Autodesk Fusion 360 part; units mm, degrees
note: some values were not read from the file. Chosen so that the rebuilt part matches the saved one: which bodies a step acts on.
(part 2 of 2)
sketch "Sketch15" plane through (0, 0, 0.1) normal (0, 0, 1) x (1, 0, 0)
  line L0 (4.15, 10.85) -> (4.15, 6.55)
  line L1 (4.15, 6.55) -> (18.55, 6.55)
  line L2 (18.55, 6.55) -> (18.55, 10.85)
  line L3 (18.55, 10.85) -> (4.15, 10.85)
  line L4 (4.7609, 8.6617) -> (4.7609, 10.2617)
  line L5 (4.7609, 10.2617) -> (5.2444, 10.2617)
  line L6 (5.2444, 10.2617) -> (5.5347, 9.1703)
  line L7 (5.5347, 9.1703) -> (5.8218, 10.2617)
  line L8 (5.8218, 10.2617) -> (6.3063, 10.2617)
  line L9 (6.3063, 10.2617) -> (6.3063, 8.6617)
  line L10 (6.3063, 8.6617) -> (6.0062, 8.6617)
  line L11 (6.0062, 8.6617) -> (6.0062, 9.9212)
  line L12 (6.0062, 9.9212) -> (5.6886, 8.6617)
  line L13 (5.6886, 8.6617) -> (5.3776, 8.6617)
  line L14 (5.3776, 8.6617) -> (5.0611, 9.9212)
  line L15 (5.0611, 9.9212) -> (5.0611, 8.6617)
  line L16 (5.0611, 8.6617) -> (4.7609, 8.6617)
  line L17 (6.6872, 9.9779) -> (6.6872, 10.2617)
  line L18 (6.6872, 10.2617) -> (6.9939, 10.2617)
  line L19 (6.9939, 10.2617) -> (6.9939, 9.9779)
  line L20 (6.9939, 9.9779) -> (6.6872, 9.9779)
  line L21 (6.6872, 8.6617) -> (6.6872, 9.8207)
  line L22 (6.6872, 9.8207) -> (6.9939, 9.8207)
  line L23 (6.9939, 9.8207) -> (6.9939, 8.6617)
  line L24 (6.9939, 8.6617) -> (6.6872, 8.6617)
  line L25 (8.381, 9.478) -> (8.0787, 9.4235)
  spline S0 degree 2 poles (8.0787, 9.4235) (8.0634, 9.5141) (8.0088, 9.5599) knots 0 0 0 1 1 1
  spline S1 degree 2 poles (8.0088, 9.5599) (7.9553, 9.6057) (7.8691, 9.6057) knots 0 0 0 1 1 1
  spline S2 degree 2 poles (7.8691, 9.6057) (7.7545, 9.6057) (7.6858, 9.5261) knots 0 0 0 1 1 1
  spline S3 degree 2 poles (7.6858, 9.5261) (7.6181, 9.4475) (7.6181, 9.2619) knots 0 0 0 1 1 1
  spline S4 degree 2 poles (7.6181, 9.2619) (7.6181, 9.0557) (7.6869, 8.9705) knots 0 0 0 1 1 1
  spline S5 degree 2 poles (7.6869, 8.9705) (7.7567, 8.8854) (7.8735, 8.8854) knots 0 0 0 1 1 1
  spline S6 degree 2 poles (7.8735, 8.8854) (7.9608, 8.8854) (8.0165, 8.9345) knots 0 0 0 1 1 1
  spline S7 degree 2 poles (8.0165, 8.9345) (8.0721, 8.9847) (8.095, 9.1059) knots 0 0 0 1 1 1
  line L26 (8.095, 9.1059) -> (8.3963, 9.0546)
  spline S8 degree 2 poles (8.3963, 9.0546) (8.3493, 8.8472) (8.2162, 8.7413) knots 0 0 0 1 1 1
  spline S9 degree 2 poles (8.2162, 8.7413) (8.083, 8.6355) (7.8593, 8.6355) knots 0 0 0 1 1 1
  spline S10 degree 2 poles (7.8593, 8.6355) (7.605, 8.6355) (7.4533, 8.7959) knots 0 0 0 1 1 1
  spline S11 degree 2 poles (7.4533, 8.7959) (7.3027, 8.9564) (7.3027, 9.2401) knots 0 0 0 1 1 1
  spline S12 degree 2 poles (7.3027, 9.2401) (7.3027, 9.5272) (7.4544, 9.6865) knots 0 0 0 1 1 1
  spline S13 degree 2 poles (7.4544, 9.6865) (7.6061, 9.8469) (7.8648, 9.8469) knots 0 0 0 1 1 1
  spline S14 degree 2 poles (7.8648, 9.8469) (8.0765, 9.8469) (8.2009, 9.7553) knots 0 0 0 1 1 1
  spline S15 degree 2 poles (8.2009, 9.7553) (8.3264, 9.6647) (8.381, 9.478) knots 0 0 0 1 1 1
  line L27 (8.9692, 8.6617) -> (8.6625, 8.6617)
  line L28 (8.6625, 8.6617) -> (8.6625, 9.8207)
  line L29 (8.6625, 9.8207) -> (8.9474, 9.8207)
  line L30 (8.9474, 9.8207) -> (8.9474, 9.6559)
  spline S16 degree 2 poles (8.9474, 9.6559) (9.0205, 9.7727) (9.0783, 9.8098) knots 0 0 0 1 1 1
  spline S17 degree 2 poles (9.0783, 9.8098) (9.1373, 9.8469) (9.2115, 9.8469) knots 0 0 0 1 1 1
  spline S18 degree 2 poles (9.2115, 9.8469) (9.3163, 9.8469) (9.4134, 9.7891) knots 0 0 0 1 1 1
  line L31 (9.4134, 9.7891) -> (9.3185, 9.5217)
  spline S19 degree 2 poles (9.3185, 9.5217) (9.241, 9.5719) (9.1744, 9.5719) knots 0 0 0 1 1 1
  spline S20 degree 2 poles (9.1744, 9.5719) (9.11, 9.5719) (9.0653, 9.5359) knots 0 0 0 1 1 1
  spline S21 degree 2 poles (9.0653, 9.5359) (9.0205, 9.501) (8.9943, 9.4082) knots 0 0 0 1 1 1
  spline S22 degree 2 poles (8.9943, 9.4082) (8.9692, 9.3154) (8.9692, 9.0197) knots 0 0 0 1 1 1
  line L32 (8.9692, 9.0197) -> (8.9692, 8.6617)
  spline S23 degree 2 poles (9.5367, 9.2576) (9.5367, 9.4104) (9.612, 9.5534) knots 0 0 0 1 1 1
  spline S24 degree 2 poles (9.612, 9.5534) (9.6873, 9.6963) (9.8248, 9.7716) knots 0 0 0 1 1 1
  spline S25 degree 2 poles (9.8248, 9.7716) (9.9634, 9.8469) (10.1337, 9.8469) knots 0 0 0 1 1 1
  spline S26 degree 2 poles (10.1337, 9.8469) (10.3967, 9.8469) (10.5648, 9.6756) knots 0 0 0 1 1 1
  spline S27 degree 2 poles (10.5648, 9.6756) (10.7329, 9.5053) (10.7329, 9.2445) knots 0 0 0 1 1 1
  spline S28 degree 2 poles (10.7329, 9.2445) (10.7329, 8.9815) (10.5626, 8.8079) knots 0 0 0 1 1 1
  spline S29 degree 2 poles (10.5626, 8.8079) (10.3934, 8.6355) (10.1359, 8.6355) knots 0 0 0 1 1 1
  spline S30 degree 2 poles (10.1359, 8.6355) (9.9765, 8.6355) (9.8314, 8.7075) knots 0 0 0 1 1 1
  spline S31 degree 2 poles (9.8314, 8.7075) (9.6873, 8.7795) (9.612, 8.9182) knots 0 0 0 1 1 1
  spline S32 degree 2 poles (9.612, 8.9182) (9.5367, 9.0579) (9.5367, 9.2576) knots 0 0 0 1 1 1
  spline S33 degree 2 poles (9.851, 9.2412) (9.851, 9.0688) (9.9329, 8.9771) knots 0 0 0 1 1 1
  spline S34 degree 2 poles (9.9329, 8.9771) (10.0147, 8.8854) (10.1348, 8.8854) knots 0 0 0 1 1 1
  spline S35 degree 2 poles (10.1348, 8.8854) (10.2548, 8.8854) (10.3356, 8.9771) knots 0 0 0 1 1 1
  spline S36 degree 2 poles (10.3356, 8.9771) (10.4174, 9.0688) (10.4174, 9.2434) knots 0 0 0 1 1 1
  spline S37 degree 2 poles (10.4174, 9.2434) (10.4174, 9.4137) (10.3356, 9.5053) knots 0 0 0 1 1 1
  spline S38 degree 2 poles (10.3356, 9.5053) (10.2548, 9.597) (10.1348, 9.597) knots 0 0 0 1 1 1
  spline S39 degree 2 poles (10.1348, 9.597) (10.0147, 9.597) (9.9329, 9.5053) knots 0 0 0 1 1 1
  spline S40 degree 2 poles (9.9329, 9.5053) (9.851, 9.4137) (9.851, 9.2412) knots 0 0 0 1 1 1
  line L33 (11.6386, 9.1823) -> (11.9529, 9.2128)
  spline S41 degree 2 poles (11.9529, 9.2128) (11.9813, 9.0546) (12.0675, 8.9804) knots 0 0 0 1 1 1
  spline S42 degree 2 poles (12.0675, 8.9804) (12.1549, 8.9062) (12.3022, 8.9062) knots 0 0 0 1 1 1
  spline S43 degree 2 poles (12.3022, 8.9062) (12.4583, 8.9062) (12.5368, 8.9716) knots 0 0 0 1 1 1
  spline S44 degree 2 poles (12.5368, 8.9716) (12.6165, 9.0382) (12.6165, 9.1266) knots 0 0 0 1 1 1
  spline S45 degree 2 poles (12.6165, 9.1266) (12.6165, 9.1834) (12.5827, 9.2227) knots 0 0 0 1 1 1
  spline S46 degree 2 poles (12.5827, 9.2227) (12.5499, 9.263) (12.467, 9.2925) knots 0 0 0 1 1 1
  spline S47 degree 2 poles (12.467, 9.2925) (12.4102, 9.3122) (12.2083, 9.3624) knots 0 0 0 1 1 1
  spline S48 degree 2 poles (12.2083, 9.3624) (11.9486, 9.4268) (11.8438, 9.5206) knots 0 0 0 1 1 1
  spline S49 degree 2 poles (11.8438, 9.5206) (11.6965, 9.6527) (11.6965, 9.8426) knots 0 0 0 1 1 1
  spline S50 degree 2 poles (11.6965, 9.8426) (11.6965, 9.9648) (11.7652, 10.0707) knots 0 0 0 1 1 1
  spline S51 degree 2 poles (11.7652, 10.0707) (11.8351, 10.1776) (11.965, 10.2333) knots 0 0 0 1 1 1
  spline S52 degree 2 poles (11.965, 10.2333) (12.0959, 10.289) (12.2804, 10.289) knots 0 0 0 1 1 1
  spline S53 degree 2 poles (12.2804, 10.289) (12.5816, 10.289) (12.7333, 10.1569) knots 0 0 0 1 1 1
  spline S54 degree 2 poles (12.7333, 10.1569) (12.8861, 10.0248) (12.8937, 9.8044) knots 0 0 0 1 1 1
  line L34 (12.8937, 9.8044) -> (12.5707, 9.7902)
  spline S55 degree 2 poles (12.5707, 9.7902) (12.5499, 9.9135) (12.4812, 9.967) knots 0 0 0 1 1 1
  spline S56 degree 2 poles (12.4812, 9.967) (12.4135, 10.0216) (12.2771, 10.0216) knots 0 0 0 1 1 1
  spline S57 degree 2 poles (12.2771, 10.0216) (12.1363, 10.0216) (12.0566, 9.9637) knots 0 0 0 1 1 1
  spline S58 degree 2 poles (12.0566, 9.9637) (12.0053, 9.9266) (12.0053, 9.8644) knots 0 0 0 1 1 1
  spline S59 degree 2 poles (12.0053, 9.8644) (12.0053, 9.8077) (12.0534, 9.7673) knots 0 0 0 1 1 1
  spline S60 degree 2 poles (12.0534, 9.7673) (12.1145, 9.716) (12.3502, 9.6603) knots 0 0 0 1 1 1
  spline S61 degree 2 poles (12.3502, 9.6603) (12.586, 9.6046) (12.6984, 9.5446) knots 0 0 0 1 1 1
  spline S62 degree 2 poles (12.6984, 9.5446) (12.8119, 9.4857) (12.8752, 9.382) knots 0 0 0 1 1 1
  spline S63 degree 2 poles (12.8752, 9.382) (12.9396, 9.2794) (12.9396, 9.1277) knots 0 0 0 1 1 1
  spline S64 degree 2 poles (12.9396, 9.1277) (12.9396, 8.9902) (12.8632, 8.8701) knots 0 0 0 1 1 1
  spline S65 degree 2 poles (12.8632, 8.8701) (12.7868, 8.7501) (12.6471, 8.6911) knots 0 0 0 1 1 1
  spline S66 degree 2 poles (12.6471, 8.6911) (12.5074, 8.6333) (12.2989, 8.6333) knots 0 0 0 1 1 1
  spline S67 degree 2 poles (12.2989, 8.6333) (11.9955, 8.6333) (11.8329, 8.773) knots 0 0 0 1 1 1
  spline S68 degree 2 poles (11.8329, 8.773) (11.6703, 8.9138) (11.6386, 9.1823) knots 0 0 0 1 1 1
  line L35 (13.9425, 9.0306) -> (14.2481, 8.9793)
  spline S69 degree 2 poles (14.2481, 8.9793) (14.1892, 8.8112) (14.0615, 8.7228) knots 0 0 0 1 1 1
  spline S70 degree 2 poles (14.0615, 8.7228) (13.9349, 8.6355) (13.7439, 8.6355) knots 0 0 0 1 1 1
  spline S71 degree 2 poles (13.7439, 8.6355) (13.4416, 8.6355) (13.2964, 8.833) knots 0 0 0 1 1 1
  spline S72 degree 2 poles (13.2964, 8.833) (13.1818, 8.9913) (13.1818, 9.2325) knots 0 0 0 1 1 1
  spline S73 degree 2 poles (13.1818, 9.2325) (13.1818, 9.5206) (13.3324, 9.6832) knots 0 0 0 1 1 1
  spline S74 degree 2 poles (13.3324, 9.6832) (13.483, 9.8469) (13.7133, 9.8469) knots 0 0 0 1 1 1
  spline S75 degree 2 poles (13.7133, 9.8469) (13.972, 9.8469) (14.1215, 9.6756) knots 0 0 0 1 1 1
  spline S76 degree 2 poles (14.1215, 9.6756) (14.271, 9.5053) (14.2645, 9.1528) knots 0 0 0 1 1 1
  line L36 (14.2645, 9.1528) -> (13.4961, 9.1528)
  spline S77 degree 2 poles (13.4961, 9.1528) (13.4994, 9.0164) (13.5704, 8.94) knots 0 0 0 1 1 1
  spline S78 degree 2 poles (13.5704, 8.94) (13.6413, 8.8647) (13.7472, 8.8647) knots 0 0 0 1 1 1
  spline S79 degree 2 poles (13.7472, 8.8647) (13.8192, 8.8647) (13.8683, 8.904) knots 0 0 0 1 1 1
  spline S80 degree 2 poles (13.8683, 8.904) (13.9174, 8.9433) (13.9425, 9.0306) knots 0 0 0 1 1 1
  spline S81 degree 2 poles (13.96, 9.3405) (13.9567, 9.4737) (13.8912, 9.5424) knots 0 0 0 1 1 1
  spline S82 degree 2 poles (13.8912, 9.5424) (13.8257, 9.6123) (13.7319, 9.6123) knots 0 0 0 1 1 1
  spline S83 degree 2 poles (13.7319, 9.6123) (13.6315, 9.6123) (13.566, 9.5392) knots 0 0 0 1 1 1
  spline S84 degree 2 poles (13.566, 9.5392) (13.5005, 9.466) (13.5016, 9.3405) knots 0 0 0 1 1 1
  line L37 (13.5016, 9.3405) -> (13.96, 9.3405)
  line L38 (14.8702, 8.6617) -> (14.5635, 8.6617)
  line L39 (14.5635, 8.6617) -> (14.5635, 9.8207)
  line L40 (14.5635, 9.8207) -> (14.8483, 9.8207)
  line L41 (14.8483, 9.8207) -> (14.8483, 9.6559)
  spline S85 degree 2 poles (14.8483, 9.6559) (14.9215, 9.7727) (14.9793, 9.8098) knots 0 0 0 1 1 1
  spline S86 degree 2 poles (14.9793, 9.8098) (15.0382, 9.8469) (15.1125, 9.8469) knots 0 0 0 1 1 1
  spline S87 degree 2 poles (15.1125, 9.8469) (15.2172, 9.8469) (15.3144, 9.7891) knots 0 0 0 1 1 1
  line L42 (15.3144, 9.7891) -> (15.2194, 9.5217)
  spline S88 degree 2 poles (15.2194, 9.5217) (15.1419, 9.5719) (15.0753, 9.5719) knots 0 0 0 1 1 1
  spline S89 degree 2 poles (15.0753, 9.5719) (15.011, 9.5719) (14.9662, 9.5359) knots 0 0 0 1 1 1
  spline S90 degree 2 poles (14.9662, 9.5359) (14.9215, 9.501) (14.8953, 9.4082) knots 0 0 0 1 1 1
  spline S91 degree 2 poles (14.8953, 9.4082) (14.8702, 9.3154) (14.8702, 9.0197) knots 0 0 0 1 1 1
  line L43 (14.8702, 9.0197) -> (14.8702, 8.6617)
  line L44 (15.8273, 8.6617) -> (15.3601, 9.8207)
  line L45 (15.3601, 9.8207) -> (15.6821, 9.8207)
  line L46 (15.6821, 9.8207) -> (15.9004, 9.2292)
  line L47 (15.9004, 9.2292) -> (15.9637, 9.0317)
  spline S92 degree 2 poles (15.9637, 9.0317) (15.9888, 9.107) (15.9953, 9.131) knots 0 0 0 1 1 1
  spline S93 degree 2 poles (15.9953, 9.131) (16.0106, 9.1801) (16.0281, 9.2292) knots 0 0 0 1 1 1
  line L48 (16.0281, 9.2292) -> (16.2486, 9.8207)
  line L49 (16.2486, 9.8207) -> (16.564, 9.8207)
  line L50 (16.564, 9.8207) -> (16.1034, 8.6617)
  line L51 (16.1034, 8.6617) -> (15.8273, 8.6617)
  spline S94 degree 2 poles (16.7429, 9.2576) (16.7429, 9.4104) (16.8182, 9.5534) knots 0 0 0 1 1 1
  spline S95 degree 2 poles (16.8182, 9.5534) (16.8935, 9.6963) (17.031, 9.7716) knots 0 0 0 1 1 1
  spline S96 degree 2 poles (17.031, 9.7716) (17.1696, 9.8469) (17.3399, 9.8469) knots 0 0 0 1 1 1
  spline S97 degree 2 poles (17.3399, 9.8469) (17.6029, 9.8469) (17.771, 9.6756) knots 0 0 0 1 1 1
  spline S98 degree 2 poles (17.771, 9.6756) (17.9391, 9.5053) (17.9391, 9.2445) knots 0 0 0 1 1 1
  spline S99 degree 2 poles (17.9391, 9.2445) (17.9391, 8.9815) (17.7688, 8.8079) knots 0 0 0 1 1 1
  spline S100 degree 2 poles (17.7688, 8.8079) (17.5997, 8.6355) (17.3421, 8.6355) knots 0 0 0 1 1 1
  spline S101 degree 2 poles (17.3421, 8.6355) (17.1827, 8.6355) (17.0376, 8.7075) knots 0 0 0 1 1 1
  spline S102 degree 2 poles (17.0376, 8.7075) (16.8935, 8.7795) (16.8182, 8.9182) knots 0 0 0 1 1 1
  spline S103 degree 2 poles (16.8182, 8.9182) (16.7429, 9.0579) (16.7429, 9.2576) knots 0 0 0 1 1 1
  spline S104 degree 2 poles (17.0572, 9.2412) (17.0572, 9.0688) (17.1391, 8.9771) knots 0 0 0 1 1 1
  spline S105 degree 2 poles (17.1391, 8.9771) (17.2209, 8.8854) (17.341, 8.8854) knots 0 0 0 1 1 1
  spline S106 degree 2 poles (17.341, 8.8854) (17.4611, 8.8854) (17.5418, 8.9771) knots 0 0 0 1 1 1
  spline S107 degree 2 poles (17.5418, 8.9771) (17.6237, 9.0688) (17.6237, 9.2434) knots 0 0 0 1 1 1
  spline S108 degree 2 poles (17.6237, 9.2434) (17.6237, 9.4137) (17.5418, 9.5053) knots 0 0 0 1 1 1
  spline S109 degree 2 poles (17.5418, 9.5053) (17.4611, 9.597) (17.341, 9.597) knots 0 0 0 1 1 1
  spline S110 degree 2 poles (17.341, 9.597) (17.2209, 9.597) (17.1391, 9.5053) knots 0 0 0 1 1 1
  spline S111 degree 2 poles (17.1391, 9.5053) (17.0572, 9.4137) (17.0572, 9.2412) knots 0 0 0 1 1 1
  line L52 (10.4517, 7.1524) -> (10.6743, 7.177)
  spline S112 degree 2 poles (10.6743, 7.177) (10.6825, 7.109) (10.7169, 7.0763) knots 0 0 0 1 1 1
  spline S113 degree 2 poles (10.7169, 7.0763) (10.7512, 7.0435) (10.8077, 7.0435) knots 0 0 0 1 1 1
  spline S114 degree 2 poles (10.8077, 7.0435) (10.8789, 7.0435) (10.9289, 7.109) knots 0 0 0 1 1 1
  spline S115 degree 2 poles (10.9289, 7.109) (10.9788, 7.1745) (10.9927, 7.3808) knots 0 0 0 1 1 1
  spline S116 degree 2 poles (10.9927, 7.3808) (10.906, 7.2801) (10.7758, 7.2801) knots 0 0 0 1 1 1
  spline S117 degree 2 poles (10.7758, 7.2801) (10.6342, 7.2801) (10.5311, 7.389) knots 0 0 0 1 1 1
  spline S118 degree 2 poles (10.5311, 7.389) (10.4287, 7.4986) (10.4287, 7.6738) knots 0 0 0 1 1 1
  spline S119 degree 2 poles (10.4287, 7.6738) (10.4287, 7.8564) (10.5368, 7.9677) knots 0 0 0 1 1 1
  spline S120 degree 2 poles (10.5368, 7.9677) (10.6457, 8.0798) (10.8135, 8.0798) knots 0 0 0 1 1 1
  spline S121 degree 2 poles (10.8135, 8.0798) (10.996, 8.0798) (11.113, 7.9382) knots 0 0 0 1 1 1
  spline S122 degree 2 poles (11.113, 7.9382) (11.2301, 7.7974) (11.2301, 7.4741) knots 0 0 0 1 1 1
  spline S123 degree 2 poles (11.2301, 7.4741) (11.2301, 7.145) (11.1081, 6.9993) knots 0 0 0 1 1 1
  spline S124 degree 2 poles (11.1081, 6.9993) (10.9862, 6.8536) (10.7905, 6.8536) knots 0 0 0 1 1 1
  spline S125 degree 2 poles (10.7905, 6.8536) (10.6497, 6.8536) (10.563, 6.9281) knots 0 0 0 1 1 1
  spline S126 degree 2 poles (10.563, 6.9281) (10.4762, 7.0034) (10.4517, 7.1524) knots 0 0 0 1 1 1
  spline S127 degree 2 poles (10.9723, 7.655) (10.9723, 7.7663) (10.9207, 7.8277) knots 0 0 0 1 1 1
  spline S128 degree 2 poles (10.9207, 7.8277) (10.8699, 7.8891) (10.8028, 7.8891) knots 0 0 0 1 1 1
  spline S129 degree 2 poles (10.8028, 7.8891) (10.739, 7.8891) (10.6964, 7.8383) knots 0 0 0 1 1 1
  spline S130 degree 2 poles (10.6964, 7.8383) (10.6547, 7.7884) (10.6547, 7.6738) knots 0 0 0 1 1 1
  spline S131 degree 2 poles (10.6547, 7.6738) (10.6547, 7.5576) (10.7005, 7.5027) knots 0 0 0 1 1 1
  spline S132 degree 2 poles (10.7005, 7.5027) (10.7463, 7.4487) (10.8151, 7.4487) knots 0 0 0 1 1 1
  spline S133 degree 2 poles (10.8151, 7.4487) (10.8814, 7.4487) (10.9264, 7.5011) knots 0 0 0 1 1 1
  spline S134 degree 2 poles (10.9264, 7.5011) (10.9723, 7.5535) (10.9723, 7.655) knots 0 0 0 1 1 1
  line L53 (11.4535, 6.8176) -> (11.7163, 6.7857)
  spline S135 degree 2 poles (11.7163, 6.7857) (11.7228, 6.7398) (11.7466, 6.7227) knots 0 0 0 1 1 1
  spline S136 degree 2 poles (11.7466, 6.7227) (11.7793, 6.6981) (11.8497, 6.6981) knots 0 0 0 1 1 1
  spline S137 degree 2 poles (11.8497, 6.6981) (11.9397, 6.6981) (11.9848, 6.7251) knots 0 0 0 1 1 1
  spline S138 degree 2 poles (11.9848, 6.7251) (12.0151, 6.7431) (12.0306, 6.7832) knots 0 0 0 1 1 1
  spline S139 degree 2 poles (12.0306, 6.7832) (12.0412, 6.8119) (12.0412, 6.8888) knots 0 0 0 1 1 1
  line L54 (12.0412, 6.8888) -> (12.0412, 7.0157)
  spline S140 degree 2 poles (12.0412, 7.0157) (11.9381, 6.8749) (11.7809, 6.8749) knots 0 0 0 1 1 1
  spline S141 degree 2 poles (11.7809, 6.8749) (11.6058, 6.8749) (11.5035, 7.0231) knots 0 0 0 1 1 1
  spline S142 degree 2 poles (11.5035, 7.0231) (11.4232, 7.1401) (11.4232, 7.3145) knots 0 0 0 1 1 1
  spline S143 degree 2 poles (11.4232, 7.3145) (11.4232, 7.533) (11.528, 7.6484) knots 0 0 0 1 1 1
  spline S144 degree 2 poles (11.528, 7.6484) (11.6336, 7.7639) (11.79, 7.7639) knots 0 0 0 1 1 1
  spline S145 degree 2 poles (11.79, 7.7639) (11.9512, 7.7639) (12.056, 7.6222) knots 0 0 0 1 1 1
  line L55 (12.056, 7.6222) -> (12.056, 7.7442)
  line L56 (12.056, 7.7442) -> (12.2713, 7.7442)
  line L57 (12.2713, 7.7442) -> (12.2713, 6.9641)
  spline S146 degree 2 poles (12.2713, 6.9641) (12.2713, 6.8102) (12.2459, 6.7341) knots 0 0 0 1 1 1
  spline S147 degree 2 poles (12.2459, 6.7341) (12.2205, 6.658) (12.1747, 6.6146) knots 0 0 0 1 1 1
  spline S148 degree 2 poles (12.1747, 6.6146) (12.1288, 6.5712) (12.0519, 6.5467) knots 0 0 0 1 1 1
  spline S149 degree 2 poles (12.0519, 6.5467) (11.9758, 6.5221) (11.8587, 6.5221) knots 0 0 0 1 1 1
  spline S150 degree 2 poles (11.8587, 6.5221) (11.6377, 6.5221) (11.5452, 6.5982) knots 0 0 0 1 1 1
  spline S151 degree 2 poles (11.5452, 6.5982) (11.4527, 6.6735) (11.4527, 6.7898) knots 0 0 0 1 1 1
  spline S152 degree 2 poles (11.4527, 6.7898) (11.4527, 6.8012) (11.4535, 6.8176) knots 0 0 0 1 1 1
  spline S153 degree 2 poles (11.659, 7.3276) (11.659, 7.1892) (11.7122, 7.1246) knots 0 0 0 1 1 1
  spline S154 degree 2 poles (11.7122, 7.1246) (11.7662, 7.0607) (11.8448, 7.0607) knots 0 0 0 1 1 1
  spline S155 degree 2 poles (11.8448, 7.0607) (11.9291, 7.0607) (11.9872, 7.1262) knots 0 0 0 1 1 1
  spline S156 degree 2 poles (11.9872, 7.1262) (12.0453, 7.1925) (12.0453, 7.3218) knots 0 0 0 1 1 1
  spline S157 degree 2 poles (12.0453, 7.3218) (12.0453, 7.4569) (11.9897, 7.5224) knots 0 0 0 1 1 1
  spline S158 degree 2 poles (11.9897, 7.5224) (11.934, 7.5879) (11.8489, 7.5879) knots 0 0 0 1 1 1
  spline S159 degree 2 poles (11.8489, 7.5879) (11.7662, 7.5879) (11.7122, 7.5232) knots 0 0 0 1 1 1
  spline S160 degree 2 poles (11.7122, 7.5232) (11.659, 7.4594) (11.659, 7.3276) knots 0 0 0 1 1 1
extrude "Extrude15" cut sketch "Sketch15" against normal blind 0.05 contours L1 L53 S135 S136 S137 S138 S139 L54 S140 S141 S142 S143 S144 S145 L55 L56 L57 S146 S147 S148 S150 S151 S152 | L4 L5 L6 L7 L8 L9 L10 L11 L12 L13 L14 L15 L16 | L17 L18 L19 L20 | L21 L22 L23 L24 | L25 S0 S1 S2 S3 S4 S5 S6 S7 L26 S8 S9 S10 S11 S12 S13 S14 S15 | L27 L28 L29 L30 S16 S17 S18 L31 S19 S20 S21 S22 L32 | S23 S24 S25 S26 S27 S28 S29 S30 S31 S32 | L33 S41 S42 S43 S44 S45 S46 S47 S48 S49 S50 S51 S52 S53 S54 L34 S55 S56 S57 S58 S59 S60 S61 S62 S63 S64 S65 S66 S67 S68 | L35 S69 S70 S71 S72 S73 S74 S75 S76 L36 S77 S78 S79 S80 | L38 L39 L40 L41 S85 S86 S87 L42 S88 S89 S90 S91 L43 | L44 L45 L46 L47 S92 S93 L48 L49 L50 L51 | S94 S95 S96 S97 S98 S99 S100 S101 S102 S103 | L52 S112 S113 S114 S115 S116 S117 S118 S119 S120 S121 S122 S123 S124 S125 S126 bodies 7
ref_plane "WorkPlane2" through (11.35, 11.15, -6.15) normal (0, 0, 1) x (1, 0, 0)
mirror "Mirror4" about plane through (11.35, 11.15, -6.15) normal (0, 0, 1) of bodies 7 makes body 8
mirror "Mirror5" about plane through (11.35, 0, 0) normal (1, 0, 0) of bodies 8 makes body 9
sketch "Sketch16" plane through (0, 0, 0) normal (-1, 0, 0) x (0, 0, 1)
  line L0 (0, 15.8) -> (-1, 15.8)
  line L1 (-1, 15.8) -> (-1, 16.8)
  line L2 (-1, 16.8) -> (-11.3, 16.8)
  line L3 (-11.3, 16.8) -> (-11.3, 15.8)
  line L4 (-11.3, 15.8) -> (-12.3, 15.8)
  line L5 (-12.3, 15.8) -> (-12.3, 0)
  line L6 (-12.3, 0) -> (0, 0)
  line L7 (0, 0) -> (0, 15.8)
  line L8 (-6.15, 0) -> (-6.15, 4.5)
  circle A0 centre (-6.15, 5) radius 0.5
  circle A1 centre (-5.15, 5) radius 0.5
  circle A2 centre (-7.15, 5) radius 0.5
  dimension "d106" = 4.5
  dimension "d107" = 1
  dimension "d108" = 1
  dimension "d109" = 1
  constraint midpoint L6 L8.start
  constraint perpendicular L6 L8
  constraint coincident L8.end A0
  measures "d106" distance of L8.start L8.end
  measures "d107" diameter of A0
  measures "d108" diameter of A1
  measures "d109" diameter of A2
extrude "Extrude16" add sketch "Sketch16" along normal blind 8 separate body contours A0 | A2 | A1 makes body 10 at (0, 4.9582, -6.9669)
hidden bodies 8
equation "d62 = ( 22.7 / 2 ) * 1 mm"
equation "d69 = ( 17 / 2 ) * 1 mm"
equation "d75 = ( 11.5 / 2 ) * 1 mm"
equation "d76 = ( 7.7 * 2 ) * 1 mm"
equation "d77 = ( 5.75 * 2 ) * 1 mm"
equation "d101 = ( -12.3 / 2 ) * 1 mm"
